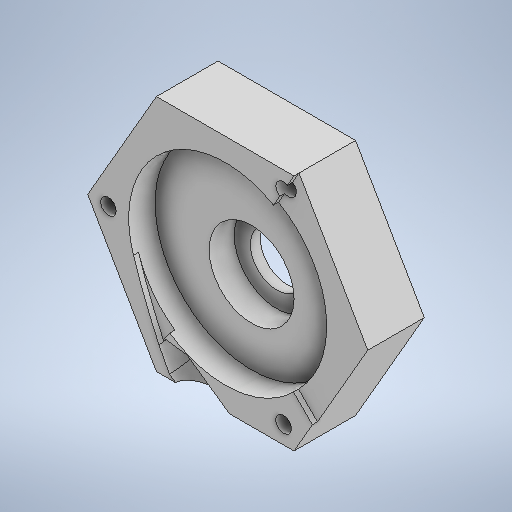
# Autodesk Inventor part: Case
Saved by Autodesk Inventor 2026.1 (Build 301233020, 233B)
## iProperties
Created: 2025-10-20
Part Number: Case
Material: Generic
Document SubType Name: Modeling
Designer: yo
Density: 1 g/cm^3
Appearance: Default
Author: yo
Autodesk Inventor part; units mm, degrees
ref_plane "YZ Plane" through (0, 0, 0) normal (1, 0, 0) x (0, 1, 0)
ref_plane "XZ Plane" through (0, 0, 0) normal (0, 1, 0) x (-1, 0, 0)
ref_plane "XY Plane" through (0, 0, 0) normal (0, 0, 1) x (1, 0, 0)
sketch "Sketch1" plane through (0, 0, 0) normal (0, 0, 1) x (1, 0, 0)
  circle A0 centre (0, 0) radius 19.2
  line L0 (-13.683201, 23.7) -> (13.683201, 23.7)
  line L1 (13.683201, 23.7) -> (27.366403, 0)
  line L2 (27.366403, 0) -> (13.683201, -23.7)
  line L3 (13.683201, -23.7) -> (-13.683201, -23.7)
  line L4 (-13.683201, -23.7) -> (-27.366403, 0)
  line L5 (-27.366403, 0) -> (-13.683201, 23.7)
  circle A1 centre (11.620726, 20.127688) radius 1.55
  line L6 (0, 23.7) -> (0, 19.2) construction
  circle A2 centre (0, -2.7) radius 5.25
  circle A3 centre (0, -2.7) radius 8.45
  line L7 (11.620726, 20.127688) -> (9.6, 16.627688) construction
  circle A4 centre (-23.241452, 0) radius 1.55
  circle A5 centre (11.620726, -20.127688) radius 1.55
  point P0 (0, 21.45)
  point P1 (0, -19.2)
  dimension "d1" = 3.1
  dimension "d2" = 4.5
  dimension "d23" = 10.5
  dimension "d24" = 16.9
  dimension "d46" = 3.5
  dimension "d47" = -30
  dimension "d50" = 360
  dimension "d53" = 16.5
  dimension "d54" = 2.7
  constraints: 16 end point, 6 centre point, 3 coincident, 3 point on circle, 2 midpoint, 2 vertical alignment, 1 horizontal, 1 line through centre, 1 vertical, 20 other
  measures "d1" diameter of A1
  measures "d2" distance of L6.start L6.end
  measures "d23" diameter of A2
  measures "d24" diameter of A3
  measures "d46" vertical distance of L7.start L7.end
  measures "d47" angle of L6 L7
  measures "d53" distance of A0.end A2.centre
  measures "d54" distance of A2.centre A0.centre
extrude "Extrusion1" add sketch "Sketch1" along normal blind 2 contours A3
extrude "Extrusion2" add sketch "Sketch1" along normal blind 7 contours A0
extrude "Extrusion3" add sketch "Sketch1" along normal blind 12.25 contours L0 L1 L2 L3 L4 L5
sketch "Sketch2" plane through (0, 0, 12.25) normal (0, 0, 1) x (1, 0, 0)
  circle A0 centre (0, 0) radius 19.2
  line L0 (0, -19.2) -> (0, -23.7) construction
  line L1 (-13.683201, -23.7) -> (13.683201, -23.7)
  line L2 (-11.012668, -15.727719) -> (-14.999056, -21.420872) construction
  line L3 (-18.260285, -5.933126) -> (-23.043597, -7.487319) construction
  line L4 (9.6, 16.627688) -> (13.683201, 23.7)
  line L5 (13.57645, -13.57645) -> (17.349604, -17.349604)
  line L6 (13.683201, -23.7) -> (27.366403, 0)
  line L7 (27.366403, 0) -> (13.683201, 23.7)
  line L8 (-27.366403, 0) -> (-13.683201, -23.7)
  circle A1 centre (0, -2.7) radius 5.25
  line L9 (-11.012668, -15.727719) -> (-13.192258, -18.840497)
  arc A2 (-18.260285, -5.933126) -> (-13.192258, -18.840497) centre (91.721489, 29.802118) ccw
  dimension "d15" = 35
  dimension "d16" = 72
  dimension "d18" = 150
  dimension "d19" = 45
  dimension "d45" = 3.8
  constraints: 12 end point, 7 point on circle, 4 line through centre, 4 point on line, 1 centre point, 1 midpoint, 1 tangent, 1 vertical
  measures "d15" angle of L0 L2
  measures "d16" angle of L0 L3
  measures "d18" angle of L4 L0
  measures "d19" angle of L0 L5
  measures "d45" distance of L9.end L2.start
extrude "Extrusion5" cut sketch "Sketch2" against normal blind 1 contours A0 L4 L7 L6 L5 | A0 L9 A2
ref_plane "Work Plane1" through (0, 0, 12.25) normal (0, 0, 1) x (1, 0, 0)
sketch "Sketch3" plane through (0, 0, 12.25) normal (0, 0, 1) x (1, 0, 0)
  line L0 (-11.012668, -15.727719) -> (-13.192258, -18.840497)
  line L1 (-12.102463, -17.284108) -> (-11.012668, -15.727719)
  line L2 (-12.618682, -18.021345) -> (7.040967, -31.787179)
  line L3 (-11.105821, -22.834543) -> (5.27722, -34.306072)
  line L4 (-11.105821, -22.834543) -> (-13.192258, -18.840497)
  line L5 (5.27722, -34.306072) -> (7.040967, -31.787179)
  point P0 (0, 0)
  point P1 (-11.586244, -16.546871)
  dimension "d36" = 6.15
  dimension "d39" = 4
  dimension "d41" = 20
  dimension "d43" = 2
  constraints: 10 end point, 2 perpendicular, 1 collinear, 1 midpoint, 1 parallel, 1 point on line
  measures "d36" diameter of L3 L2
  measures "d39" distance from line of L3.start L0
  measures "d41" distance of L3.start L3.end
  measures "d43" diameter of L0.end L2
revolve "Revolution1" cut sketch "Sketch3" angle 360 about axis through (-12.618682, -18.021345, 12.25) along (0.819152, -0.5735764, 0)
body "Solid1"
